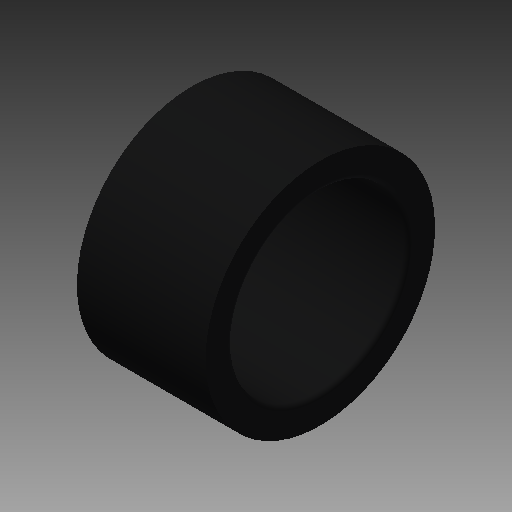
# Autodesk Inventor part: HSK-K 1.209.1201.70-Sealing insert
Saved by Autodesk Inventor 2018 (Build 220112000, 112)
## iProperties
Category: PARTsolutions
Company: SEALCON
Created: 2018-02-18
Part Number: HSK-K 1.209.1201.70-Sealing insert
Catalog Web Link: www.cadenas.de
Description: HSK-K NPT-Sealing insert-Industrial cable glands
Vendor: SEALCON
Document SubType Name: Modeling
Designer: psAdmin
Manufacturer: SEALCON
Mass: 0.707624 g
Surface Area: 9.21971 cm^2
Volume: 0.707624 cm^3
Density: 1 g/cm^3
Material: Generic
Appearance: PSOLRGB-10-10-10
PSOL_IDENT_0: {$CADENAS_DATA\23d-libs\sealcon\kabelverschraubungen\industriekabelverschraubungen\hsk_standard_kabe
PSOL_IDENT_1: lver\hsk_k\npt\hsk_k_npt_seal_insert.prj},242 {VTYP=3D},{NB=HSK-K 1.209.1201.70-Sealing insert},{LIN
PSOL_IDENT_2: A=HSK-K 1.209.1201.70-Sealing insert},{NN=HSK-K NPT-Sealing insert},{DATE=25.01.2018 07:57:44},{GEOM
PSOL_IDENT_3: DATE=03.03.2011 00:00:00},{VERSION=v110309072932},{LINEID=200},{LINESUBID=-1},{WBVAR=}  {NB=HSK-K 1.
PSOL_IDENT_4: 209.1201.70_sealing insert},{LINA=HSK-K 1.209.1201.70_sealing insert},{KT=DUMMY},{AG=1/2\" NPT},{FR=
PSOL_IDENT_5: black},{GL=13},{H=27},{SW=24},{BN=1.209.1201.70},{COLX=0.04,0.04,0.04,0.00},{VER=3}
NN: HSK-K NPT-Sealing insert
NT: Industrial cable glands
NB: HSK-K 1.209.1201.70-Sealing insert
NBSYN: HSK-K $BN.-Sealing insert
LINA: HSK-K 1.209.1201.70-Sealing insert
AG: 1/2" NPT
FR: black
GL: 13
H: 27
SW: 24
BN: 1.209.1201.70
VER: 3
SUPPLIER: SEALCON
ARTICLENO: HSK-K 1.209.1201.70-Sealing insert
BOMINFO: HSK-K 1.209.1201.70-Sealing insert
CREATOR: CADENAS GmbH
Title: HSK-K 1.209.1201.70-Sealing insert
Author: Cadenas PARTsolutions
Comments: Industrial cable glands
Autodesk Inventor part; units mm, degrees
sketch "Sketch_1" plane through (0, 0, 0) normal (0, 0, 1) x (1, 0, 0)
  line L0 (10.8, 0) -> (0, 0)
  line L1 (2, 6) -> (10.5, 6)
  arc A0 (10.5, 6) -> (10.8, 6.3) centre (10.5, 6.3) ccw
  line L2 (10.8, 6.3) -> (10.8, 7.85)
  line L3 (10.8, 7.85) -> (2, 7.85)
  line L4 (2, 7.85) -> (2, 6)
  constraints: 10 end point, 2 point on circle, 1 centre point
revolve "Revolution1" add sketch "Sketch_1" angle 360 about axis through (10.8, 0, 0) along (1, 0, 0)
ref_plane "IP1_XY" through (0, 0, 0) normal (1, 0, 0) x (0, 0, -1)
ref_plane "IP1_YZ" through (0, 0, 0) normal (0, 0, -1) x (0, 1, 0)
ref_plane "IP1_ZX" through (0, 0, 0) normal (0, 1, 0) x (1, 0, 0)
body "Solid1"
